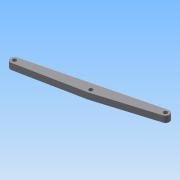
# Autodesk Inventor part: 1-2
Saved by Autodesk Inventor 2015 (Build 190159000, 159)
## iProperties
Created: 2018-05-07
Part Number: 1-2
Material: 一般
Document SubType Name: Modeling
Designer: 王博聖
Density: 1 g/cm^3
Appearance: 預設
Author: 王博聖
Autodesk Inventor part; units mm, degrees
ref_plane "YZ Plane" through (0, 0, 0) normal (1, 0, 0) x (0, 1, 0)
ref_plane "XZ Plane" through (0, 0, 0) normal (0, 1, 0) x (-1, 0, 0)
ref_plane "XY Plane" through (0, 0, 0) normal (0, 0, 1) x (1, 0, 0)
sketch "草圖1" plane through (0, 0, 0) normal (0, 0, 1) x (1, 0, 0)
  line L0 (0, 0) -> (-20.4461, -4.0839) construction
  line L1 (-20.4461, -4.0839) -> (18.3584, 5.6222) construction
  line L2 (18.3584, 5.6222) -> (0, 0) construction
  line L3 (-20.4461, -4.0839) -> (18.3584, 5.6222) construction
  line L4 (-20.1428, -5.2965) -> (18.6617, 4.4095)
  line L5 (18.0551, 6.8348) -> (-20.7494, -2.8712)
  arc A0 (-20.7494, -2.8712) -> (-20.1428, -5.2965) centre (-20.4461, -4.0839) ccw
  arc A1 (18.6617, 4.4095) -> (18.0551, 6.8348) centre (18.3584, 5.6222) ccw
  line L6 (0, 0) -> (-20.4461, -4.0839) construction
  line L7 (-0.2448, 1.2258) -> (-20.691, -2.8581)
  line L8 (-20.2013, -5.3097) -> (0.2448, -1.2258)
  arc A2 (0.2448, -1.2258) -> (-0.2448, 1.2258) centre (0, 0) ccw
  arc A3 (-20.691, -2.8581) -> (-20.2013, -5.3097) centre (-20.4461, -4.0839) ccw
  line L9 (0, 0) -> (18.3584, 5.6222) construction
  line L10 (0.366, -1.1952) -> (18.7244, 4.427)
  line L11 (17.9924, 6.8174) -> (-0.366, 1.1952)
  arc A4 (-0.366, 1.1952) -> (0.366, -1.1952) centre (0, 0) ccw
  arc A5 (18.7244, 4.427) -> (17.9924, 6.8174) centre (18.3584, 5.6222) ccw
  point P0 (-1.0439, 0.7692)
  point P1 (-10.2231, -2.0419)
  point P2 (9.1792, 2.8111)
  dimension "d0" = 20.85
  dimension "d1" = 40
  dimension "d2" = 19.2
  dimension "d3" = 2.5
  dimension "d4" = 2.5
  dimension "d5" = 2.5
  constraints: 30 end point, 12 point on circle, 12 tangent, 6 centre point, 6 equal length, 3 midpoint, 2 concentric
  measures "d0" distance of L0.start L0.end
  measures "d1" distance of L0.end L1.end
  measures "d2" distance of L1.end L0.start
  measures "d3" diameter of A1
  measures "d4" diameter of A3
  measures "d5" diameter of A5
extrude "擠出1" add sketch "草圖1" along normal blind 2
sketch "草圖2" plane through (0, 0, 2) normal (0, 0, 1) x (1, 0, 0)
  arc A0 (18.7244, 4.427) -> (18.0551, 6.8348) centre (18.3584, 5.6222) ccw projected
  arc A1 (-20.7494, -2.8712) -> (-20.2013, -5.3097) centre (-20.4461, -4.0839) ccw projected
  arc A2 (0.2448, -1.2258) -> (0.366, -1.1952) centre (0, 0) ccw projected
  circle A3 centre (0, 0) radius 0.625
  circle A4 centre (18.3584, 5.6222) radius 0.625
  circle A5 centre (-20.4461, -4.0839) radius 0.625
  dimension "d8" = 1.25
  dimension "d9" = 1.25
  dimension "d10" = 1.25
  constraints: 3 centre point, 3 coincident
  measures "d8" diameter of A3
  measures "d9" diameter of A4
  measures "d10" diameter of A5
extrude "擠出2" cut sketch "草圖2" against normal blind 2
